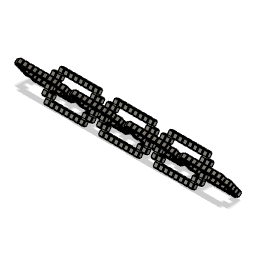
Chain v1 (Autodesk Fusion 360 design; units mm, degrees)
Autodesk Fusion 360 part; units mm, degrees
sketch "Sketch1" plane through (0, 0, 0) normal (0, 1, 0) x (1, 0, 0)
  line L0 (0, 0) -> (2.5, 0)
  line L1 (2.5, 0) -> (2.5, -2.5)
  line L2 (2.5, -2.5) -> (0, -2.5)
  line L3 (0, -2.5) -> (0, 0)
  line L4 (3, -3) -> (-0.5, -3)
  line L5 (-0.5, -3) -> (-0.5, 0.5)
  line L6 (-0.5, 0.5) -> (3, 0.5)
  line L7 (3, 0.5) -> (3, -3)
  dimension "d1" = 2.5
  dimension "d2" = 0.5
  constraint horizontal L0
  constraint vertical L1
  constraint horizontal L2
  constraint vertical L3
  constraint coincident L0.start L3.end
  constraint equal L0 L3
  constraint horizontal L4
  constraint vertical L5
  constraint horizontal L6
  constraint vertical L7
  constraint equal L5 L6
  measures "d1" distance of L1 L3
  measures "d2" distance of L1 L7
extrude "Extrude1" add sketch "Sketch1" along normal blind 2.5 contours L0 L1 L2 L3 makes body 1
extrude "Extrude2" add 1 faces at (0.8333, 0, 0.8333) along direction (0, -1, 0) blind 0.5 separate body on bodies 1 makes body 2
extrude "Extrude3" add 1 faces at (1.6667, 0.8333, 2.5) along direction (0, 0, 1) blind 0.5 separate body on bodies 1 makes body 3
extrude "Extrude4" add 1 faces at (2.5, 0.8333, 0.8333) along direction (1, 0, 0) blind 0.5 separate body on bodies 1 makes body 4
extrude "Extrude5" add 1 faces at (0.8333, 0.8333, 0) along direction (0, 0, -1) blind 0.5 separate body on bodies 1 makes body 5
extrude "Extrude6" add 1 faces at (0, 0.8333, 1.6667) along direction (-1, 0, 0) blind 0.5 separate body on bodies 1 makes body 6
extrude "Extrude7" add 1 faces at (0.8333, 2.5, 0.8333) along direction (0, 1, 0) blind 0.5 separate body on bodies 1 makes body 7
combine "Combine1" operation add target body 1 tool bodies 2 7 4 5 6 3
copy_body "CopyPasteBodies1" bodies 1 makes body 8
move_body "Move1" bodies 8 to x (1, 0, 0) y (0, 1, 0) z (0, 0, 1) at (3.5, 0, 0)
copy_body "CopyPasteBodies2" bodies 8 makes body 9
move_body "Move2" bodies 9 to x (1, 0, 0) y (0, 1, 0) z (0, 0, 1) at (3.5, 0, 0)
copy_body "CopyPasteBodies3" bodies 9 makes body 10
move_body "Move3" bodies 10 to x (1, 0, 0) y (0, 1, 0) z (0, 0, 1) at (3.5, 0, 0)
copy_body "CopyPasteBodies4" bodies 10 makes body 11
move_body "Move4" bodies 11 to x (1, 0, 0) y (0, 1, 0) z (0, 0, 1) at (0, 0, -3.5)
copy_body "CopyPasteBodies5" bodies 11 makes body 12
move_body "Move5" bodies 12 to x (1, 0, 0) y (0, 1, 0) z (0, 0, 1) at (3.5, 0, 0)
copy_body "CopyPasteBodies6" bodies 12 makes body 13
move_body "Move6" bodies 13 to x (1, 0, 0) y (0, 1, 0) z (0, 0, 1) at (0, 0, -3.5)
copy_body "CopyPasteBodies7" bodies 12 13 makes body 14 makes body 15
move_body "Move7" bodies 14 15 to x (1, 0, 0) y (0, 1, 0) z (0, 0, 1) at (0, 0, -7)
copy_body "CopyPasteBodies8" bodies 15 makes body 16
move_body "Move8" bodies 16 to x (1, 0, 0) y (0, 1, 0) z (0, 0, 1) at (-3.5, 0, 0)
copy_body "CopyPasteBodies10" bodies 1 8 10 9 makes body 17 makes body 18 makes body 19 makes body 20
move_body "Move10" bodies 17 18 19 20 to x (1, 0, 0) y (0, 1, 0) z (0, 0, 1) at (0, 0, -21)
move_body "Move11" bodies 17 18 19 20 to x (1, 0, 0) y (0, 1, 0) z (0, 0, 1) at (0, 0, 3.5)
copy_body "CopyPasteBodies11" bodies 17 18 19 20 makes body 21 makes body 22 makes body 23 makes body 24
move_body "Move12" bodies 21 22 23 24 to x (1, 0, 0) y (0, 1, 0) z (0, 0, 1) at (-14, 0, 0)
copy_body "CopyPasteBodies12" bodies 1 10 8 9 makes body 25 makes body 26 makes body 27 makes body 28
move_body "Move13" bodies 25 26 27 28 to x (1, 0, 0) y (0, 1, 0) z (0, 0, 1) at (-14, 0, 0)
copy_body "CopyPasteBodies13" bodies 11 16 makes body 29 makes body 30
move_body "Move14" bodies 29 30 to x (1, 0, 0) y (0, 1, 0) z (0, 0, 1) at (-24.5, 0, 0)
copy_body "CopyPasteBodies14" bodies 12 15 13 14 makes body 31 makes body 32 makes body 33 makes body 34
move_body "Move15" bodies 31 32 33 34 to x (1, 0, 0) y (0, 1, 0) z (0, 0, 1) at (-31.5, 0, 0)
combine "Combine2" operation add target body 1 tool bodies 16 21 23 15 22 26 18 25 28 30 29 19 31 32 33 34 20 24 27 17 13 14 10 8 9 11 12
copy_body "CopyPasteBodies17" bodies 1 makes body 35
move_body "Move20" bodies 35 to x (1, 0, 0) y (0, 0, 1) z (0, -1, 0) at (0, -14.5, -14.5)
move_body "Move21" bodies 35 to x (1, 0, 0) y (0, 1, 0) z (0, 0, 1) at (0, 0, 5.5)
move_body "Move22" bodies 35 to x (1, 0, 0) y (0, 1, 0) z (0, 0, 1) at (0, 8.5, 0)
move_body "Move23" bodies 35 to x (1, 0, 0) y (0, 1, 0) z (0, 0, 1) at (19.25, 0, 0)
copy_body "CopyPasteBodies18" bodies 35 makes body 36
move_body "Move24" bodies 36 to x (1, 0, 0) y (0, 1, 0) z (0, 0, 1) at (-38.5, 0, 0)
copy_body "CopyPasteBodies19" bodies 36 makes body 37
move_body "Move25" bodies 37 to x (1, 0, 0) y (0, 1, 0) z (0, 0, 1) at (57.75, 0, 0)
move_body "Move26" bodies 37 to x (1, 0, 0) y (0, 1, 0) z (0, 0, 1) at (19.25, 0, 0)
copy_body "CopyPasteBodies20" bodies 1 makes body 38
move_body "Move27" bodies 38 to x (1, 0, 0) y (0, 1, 0) z (0, 0, 1) at (38.5, 0, 0)
copy_body "CopyPasteBodies21" bodies 37 38 makes body 39 makes body 40
move_body "Move28" bodies 39 40 to x (1, 0, 0) y (0, 1, 0) z (0, 0, 1) at (38.5, 0, 0)
move_body "Move29" bodies 36 38 40 35 37 39 1 to x (1, 0, 0) y (0, 0.707107, 0.707107) z (0, -0.707107, 0.707107) at (0, -3.6569, -3.1716)
move_body "Move30" bodies 36 35 37 39 to x (1, 0, 0) y (0, 0.984808, -0.173648) z (0, 0.173648, 0.984808) at (0, 1.2595, 0.9821)
move_body "Move31" bodies 1 38 40 to x (1, 0, 0) y (0, 0.984808, 0.173648) z (0, -0.173648, 0.984808) at (0, -1.1021, -0.8176)
move_body "Move32" bodies 1 38 40 to x (1, 0, 0) y (0, 1, 0) z (0, 0, 1) at (0, 0, 1)
named bodies: "a1", "Cube", "Cube (1)", "Cube (1) (1)", "6 (1)", "10", "4 (1)", "11", "12", "13", "14", "11 (1)", "12 (1)", "13 (1)", "14 (1)", "1 (1)", "4 (2)", "2 (1)", "3 (1)", "5 (1)", "10 (1)", "6 (2)", "9 (1)", "7 (1)", "8 (1)", "component", "b2", "component (1)", "b1", "component (1) (1)", "b3", "component (2)", "a2", "component (1) (1) (1)", "component (2) (1)", "b4", "a3"
